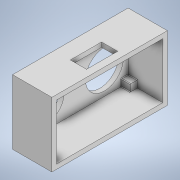
# Autodesk Inventor part: gehaeuse_hc-sr04
Saved by Autodesk Inventor 2020 (Build 240168000, 168)
## iProperties
Created: 2020-05-23
Part Number: gehaeuse_hc-sr04
Material: Generisch
Document SubType Name: Modeling
Designer: chris
Density: 1 g/cm^3
Appearance: Vorgabe
Author: chris
Autodesk Inventor part; units mm, degrees
ref_plane "YZ Plane" through (0, 0, 0) normal (1, 0, 0) x (0, 1, 0)
ref_plane "XZ Plane" through (0, 0, 0) normal (0, 1, 0) x (-1, 0, 0)
ref_plane "XY Plane" through (0, 0, 0) normal (0, 0, 1) x (1, 0, 0)
sketch "Skizze1" plane through (0, 0, 0) normal (1, 0, 0) x (0, 1, 0)
  line L0 (0, 0) -> (28, 0)
  line L1 (28, 0) -> (28, -50)
  line L2 (28, -50) -> (0, -50)
  line L3 (0, -50) -> (0, 0)
  dimension "d0" = 28
  dimension "d1" = 50
  constraints: 8 end point, 2 parallel, 1 horizontal, 1 perpendicular
  measures "d0" distance of L0.start L0.end
  measures "d1" distance of L2.end L0.start
extrude "Extrusion1" add sketch "Skizze1" along normal blind 17
shell "Wandung1" thickness 2 removed faces 1 at (17, 9.3333, -16.6667)
sketch "Skizze2" plane through (2, 2, -2) normal (1, 0, 0) x (0, 0, -1)
  circle A0 centre (35.75, 10.2) radius 8.2
  circle A1 centre (10.15, 10.2) radius 8.2
  line L0 (46, 0) -> (0, 0) projected
  line L1 (0, 0) -> (0, 24) projected
  point P0 (-2, -2)
  dimension "d5" = 16.4
  dimension "d9" = 25.6
  dimension "d10" = 10.15
  dimension "d11" = 10.2
  constraints: 2 centre point, 1 equal radius, 1 horizontal alignment
  measures "d5" diameter of A1
  measures "d9" distance of A0.centre A1.centre
  measures "d10" distance from line of A1.centre L1
  measures "d11" distance from line of L0 A0.centre
extrude "Extrusion2" cut sketch "Skizze2" against normal blind 14
sketch "Skizze3" plane through (2, 2, -2) normal (1, 0, 0) x (0, 0, -1)
  line L0 (0, 24) -> (0, 0) projected
  line L1 (0, 0) -> (3, 0)
  line L2 (3, 0) -> (3, 3)
  line L3 (3, 3) -> (0, 3)
  line L4 (0, 3) -> (0, 0)
  line L5 (0, 0) -> (46, 0) projected
  line L6 (46, 0) -> (43, 0)
  line L7 (43, 0) -> (43, 3)
  line L8 (43, 3) -> (46, 3)
  line L9 (46, 3) -> (46, 0)
  line L10 (46, 0) -> (46, 24) projected
  line L11 (46, 20) -> (43, 20)
  line L12 (43, 20) -> (43, 17)
  line L13 (43, 17) -> (46, 17)
  line L14 (46, 17) -> (46, 20)
  line L15 (0, 20) -> (3, 20)
  line L16 (3, 20) -> (3, 17)
  line L17 (3, 17) -> (0, 17)
  line L18 (0, 17) -> (0, 20)
  point P0 (-2, -2)
  point P1 (43, 0)
  point P2 (0, 20)
  point P3 (0, 17)
  dimension "d14" = 3
  dimension "d15" = 3
  dimension "d16" = 3
  dimension "d17" = 3
  dimension "d18" = 3
  dimension "d19" = 20
  constraints: 32 end point, 8 parallel, 6 point on line, 4 horizontal, 4 perpendicular
  measures "d14" distance between parallel lines of L15 L17
  measures "d15" distance between parallel lines of L0 L16
  measures "d16" distance between parallel lines of L10 L12
  measures "d17" distance between parallel lines of L5 L8
  measures "d18" distance between parallel lines of L1 L3
  measures "d19" distance between parallel lines of L15 L1
extrude "Extrusion3" add sketch "Skizze3" along normal blind 4
fillet "Rundung1" radius 0.3 23 edges at (4, 19, -5) (4, 22, -5) (4, 19, -2) (4, 22, -2) (4, 5, -2) (4, 5, -5) (4, 2, -5) (4, 22, -45) (2, 3.5, -45) (2, 5, -46.5) (4, 5, -45) (2, 22, -3.5) (2, 20.5, -5) (2, 5, -3.5) (2, 3.5, -5) (4, 19, -45) (4, 22, -48) (4, 5, -48) (4, 2, -45) (2, 22, -46.5) (2, 20.5, -45) (2, 19, -46.5) (2, 19, -3.5)
sketch "Skizze4" plane through (2, 26, -48) normal (0, -1, 0) x (1, 0, 0)
  line L0 (12, 30) -> (5, 30)
  line L1 (5, 30) -> (5, 16.5)
  line L2 (5, 16.5) -> (12, 16.5)
  line L3 (12, 16.5) -> (12, 30)
  line L4 (4, 43.3) -> (4, 45.7) projected
  line L5 (0, 46) -> (15, 46) projected
  point P0 (-2, 48)
  dimension "d23" = 1
  dimension "d24" = 7
  dimension "d25" = 13.5
  dimension "d26" = 16
  constraints: 8 end point, 2 parallel, 1 horizontal, 1 perpendicular
  measures "d23" distance between parallel lines of L1 L4
  measures "d24" distance between parallel lines of L3 L1
  measures "d25" distance between parallel lines of L2 L0
  measures "d26" distance between parallel lines of L5 L0
extrude "Extrusion4" cut sketch "Skizze4" against normal blind 17
